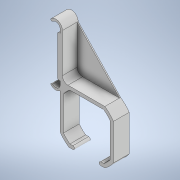
# Autodesk Inventor part: Daiso Phone Printer Adapter
Saved by Autodesk Inventor 2021 (Build 250183000, 183)
## iProperties
Created: 2021-12-02
Part Number: Daiso Phone Printer Adapter
Material: Generic
Document SubType Name: Modeling
Designer: Andrew
Density: 1 g/cm^3
Appearance: Default
Author: Andrew
Autodesk Inventor part; units mm, degrees
ref_plane "YZ Plane" through (0, 0, 0) normal (1, 0, 0) x (0, 1, 0)
ref_plane "XZ Plane" through (0, 0, 0) normal (0, 1, 0) x (-1, 0, 0)
ref_plane "XY Plane" through (0, 0, 0) normal (0, 0, 1) x (1, 0, 0)
sketch "Sketch1" plane through (0, 0, 0) normal (0, 0, 1) x (1, 0, 0)
  line L0 (-15.3704, -21.125) -> (-12.625, -21.125)
  line L1 (0, 21.125) -> (-15.3704, 21.125)
  line L2 (-21.125, 15.3704) -> (-21.125, -15.3704)
  arc A0 (-15.3704, 21.125) -> (-21.125, 15.3704) centre (0, 0) ccw
  arc A1 (-21.125, -15.3704) -> (-15.3704, -21.125) centre (0, 0) ccw
  line L3 (0, 21.125) -> (0, 24.125)
  line L4 (0, 24.125) -> (-16.3172, 24.125)
  arc A2 (-16.3172, 24.125) -> (-24.125, 16.3172) centre (0, 0) ccw
  line L5 (-24.125, 16.3172) -> (-24.125, -16.3172)
  arc A3 (-24.125, -16.3172) -> (-16.3172, -24.125) centre (0, 0) ccw
  line L6 (-16.3172, -24.125) -> (-12.625, -24.125)
  arc A4 (-12.625, -24.125) -> (-12.625, -21.125) centre (-12.625, -22.625) ccw
  line L7 (-26.625, 42.6643) -> (-26.625, 23.9143)
  line L8 (-26.625, 23.9143) -> (-24.125, 23.9143)
  line L9 (-24.125, 23.9143) -> (-24.125, 20.7893)
  arc A5 (-30.9534, 17.9609) -> (-24.125, 20.7893) centre (-28.125, 20.7893) ccw
  arc A6 (-30.9534, 17.9609) -> (-32.3676, 16.5467) centre (-31.6605, 17.2538) ccw
  arc A7 (-32.3676, 16.5467) -> (-22.125, 20.7893) centre (-28.125, 20.7893) ccw
  line L10 (-31.6605, 17.2538) -> (-28.125, 20.7893) construction
  line L11 (-26.625, 42.6643) -> (-22.125, 42.6643)
  line L12 (-22.125, 42.6643) -> (-22.125, 20.7893)
  line L13 (-16.3172, 24.125) -> (-22.125, 24.125)
  line L14 (-22.125, 42.6643) -> (-22.125, 64.5393)
  line L15 (-22.125, 64.5393) -> (16.3172, 24.125)
  line L16 (16.3172, 24.125) -> (0, 24.125)
  point P0 (-22.6762, 18.2771)
  dimension "d2" = 42.25
  dimension "d3" = 26.125
  dimension "d5" = 21.125
  dimension "d6" = 3
  dimension "d7" = 3
  dimension "d8" = 3
  dimension "d9" = 3
  dimension "d10" = 3
  dimension "d11" = 10
  dimension "d12" = 45
  dimension "d13" = 18.75
  dimension "d14" = 25.875
  dimension "d15" = 4
  dimension "d17" = 2
  dimension "d18" = 2.5
  dimension "d21" = 21.125
  dimension "d33" = 16.3172
  dimension "d34" = 16.3172
  dimension "d35" = 21.875
  dimension "d36" = 21.875
  constraints: 34 end point, 17 point on circle, 8 centre point, 7 tangent, 6 perpendicular, 5 vertical, 3 concentric, 3 horizontal, 1 coincident, 1 collinear, 1 parallel, 1 point on line, 1 vertical alignment
  measures "d2" distance between parallel lines of L0 L1
  measures "d3" radius of A1
  measures "d5" distance from line of point (0, 0) L1
  measures "d6" distance between parallel lines of L1 L4
  measures "d7" distance between parallel lines of L5 L2
  measures "d8" distance between parallel lines of L6 L0
  measures "d9" radial gap between concentric circles of A2 A0
  measures "d10" radial gap between concentric circles of A1 A3
  measures "d12" angle of L9 L10
  measures "d13" distance of L7.start L7.end
  measures "d15" radius of A5
  measures "d17" distance between parallel lines of L12 L9
  measures "d18" distance of L7.end L8.end
  measures "d21" horizontal distance of point (0, 0) L2.start
  measures "d33" distance of L3.end L4.end
  measures "d34" distance of L15.end L3.end
  measures "d35" distance of L11.end L14.end
  measures "d36" distance of L11.end L12.end
extrude "Extrusion1" add sketch "Sketch1" along normal blind 14.25 contours L0 A4 L6 A3 L5 A7 A2 L4 L3 L1 A0 L2 A1 | A2 A7
mirror "Mirror1" about plane through (0, 0, 0) normal (1, 0, 0)
extrude "Extrusion2" add sketch "Sketch1" along normal blind 14.25 separate body contours A7 A6 A5 L9 L8 L7 L11 L12 A2 | A2 A7
chamfer "Chamfer1" distance 1 angle 45 1 edges at (-26.625, 23.9143, 7.125)
mirror "Mirror2" about plane through (-22.125, 42.6643, 0) normal (0, 1, 0) bodies 2
extrude "Extrusion3" add sketch "Sketch1" along normal blind 1 contours L4 L13 L12 L14 L15 L16 bodies 2
extrude "Extrusion4" add sketch "Sketch1" along normal blind 14.25 contours A7 L12 L13 A2 bodies 2
combine bodies "Combine1" operation type add bodies to combine 2 1
fillet "Fillet1" radius 5 1 edges at (-22.125, 24.125, 7.625)
equation "\"d2\" = d0"
equation "\"d5\" = 0.5 * d2"
equation "\"d7\" = d6"
equation "\"d8\" = d6"
equation "\"d9\" = d6"
equation "\"d10\" = d6"
equation "\"d21\" = 0.5 * d0"
equation "\"d34\" = d33"
equation "\"d35\" = d36"
equation "\"d22\" = d19"
equation "\"d31\" = d19"
equation "\"d0\" = 42.25"
equation "\"d19\" = 14.25"
body "Solid1"
